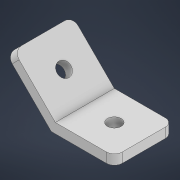
# Autodesk Inventor part: 45 degree inside coner bracket
Saved by Autodesk Inventor 2022 (Build 260153000, 153)
## iProperties
Created: 2022-01-17
Part Number: 45 degree inside coner bracket
Material: Generic
Document SubType Name: Modeling
Designer: izack
Density: 1 g/cm^3
Appearance: Default
Author: izack
Autodesk Inventor part; units mm, degrees
ref_plane "YZ Plane" through (0, 0, 0) normal (1, 0, 0) x (0, 1, 0)
ref_plane "XZ Plane" through (0, 0, 0) normal (0, 1, 0) x (-1, 0, 0)
ref_plane "XY Plane" through (0, 0, 0) normal (0, 0, 1) x (1, 0, 0)
sketch "Sketch1" plane through (0, 0, 0) normal (0, 0, 1) x (1, 0, 0)
  line L0 (0, 0) -> (15, 0)
  line L1 (0, 0) -> (-10.6066, 10.6066)
  line L2 (0, 0) -> (15, 0) construction
  line L3 (-10.6066, 10.6066) -> (-12.3744, 8.8388)
  line L4 (15, 0) -> (15, -2.5)
  line L5 (0, 0) -> (2.3007, 5.5544) construction
  line L6 (0, 0) -> (6.0121, 0) construction
  line L7 (2.3007, 5.5544) -> (-1.6655, -4.021) construction
  line L8 (-12.3744, 8.8388) -> (-1.0355, -2.5)
  line L9 (15, -2.5) -> (-1.0355, -2.5)
  dimension "d2" = 15
  dimension "d3" = 15
  dimension "d4" = 135
  dimension "d5" = 2.5
  dimension "d6" = 2.5
  dimension "d7" = 67.5
  constraints: 20 end point, 4 horizontal, 2 equal length, 2 perpendicular, 2 point on line
  measures "d2" distance of L0.start L0.end
  measures "d3" distance of L0.start L1.end
  measures "d4" angle of L2 L1
  measures "d5" distance of L1.end L3.end
  measures "d6" distance of L2.end L4.end
  measures "d7" angle of L6 L5
extrude "Extrusion1" add sketch "Sketch1" along normal blind 15
sketch "Sketch2" plane through (-10.6066, 10.6066, 0) normal (0.7071, 0.7071, 0) x (-0.7071, 0.7071, 0)
  circle A0 centre (-7.5, 7.5) radius 1.75
  line L0 (-15, 15) -> (0, 15) projected
  line L1 (-15, 0) -> (-15, 15) projected
  dimension "d10" = 3.5
  dimension "d11" = 7.5
  dimension "d12" = 7.5
  constraints: 1 centre point
  measures "d10" diameter of A0
  measures "d11" distance from line of L0 A0.centre
  measures "d12" distance from line of L1 A0.centre
sketch "Sketch3" plane through (0, 0, 0) normal (0, 1, 0) x (1, 0, 0)
  circle A0 centre (7.5, -7.5) radius 1.75
  line L0 (15, 0) -> (15, -15) projected
  line L1 (15, 0) -> (0, 0) projected
  dimension "d13" = 3.5
  dimension "d14" = 7.5
  dimension "d15" = 7.5
  constraints: 1 centre point
  measures "d13" diameter of A0
  measures "d14" distance from line of L0 A0.centre
  measures "d15" distance from line of L1 A0.centre
extrude "Extrusion2" cut sketch "Sketch2" against normal blind 15
extrude "Extrusion3" cut sketch "Sketch3" against normal blind 15
fillet "Fillet1" radius 2 4 edges at (-11.4905, 9.7227, 15) (-11.4905, 9.7227, 0) (15, -1.25, 0) (15, -1.25, 15)
body "Solid1"
